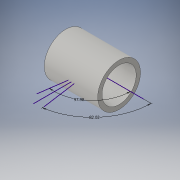
# Autodesk Inventor part: upper_arm_004
Saved by Autodesk Inventor 2016 SP1 (Build 200210100, 210)
## iProperties
Created: 2016-06-15
Part Number: upper_arm_004
Material: Generic
Document SubType Name: Modeling
Designer: asvsf
Density: 1 g/cm^3
Appearance: Default
Author: asvsf
Autodesk Inventor part; units mm, degrees
ref_plane "YZ Plane" through (0, 0, 0) normal (1, 0, 0) x (0, 1, 0)
ref_plane "XZ Plane" through (0, 0, 0) normal (0, 1, 0) x (-1, 0, 0)
ref_plane "XY Plane" through (0, 0, 0) normal (0, 0, 1) x (1, 0, 0)
sketch "Sketch1" plane through (0, 0, 0) normal (1, 0, 0) x (0, 1, 0)
  circle A0 centre (0, 0) radius 20
  circle A1 centre (0, 0) radius 16
  dimension "d0" = 40
  dimension "d1" = 32
  constraints: 2 centre point, 2 coincident
  measures "d0" diameter of A0
  measures "d1" diameter of A1
extrude "Extrusion1" add sketch "Sketch1" along normal mid plane 50
sketch "Sketch2" plane through (0, 0, 0) normal (0, 1, 0) x (-1, 0, 0)
  line L0 (0, 0) -> (6.4421, 45.9543)
  line L1 (0, 0) -> (-47.755, 0)
  line L2 (0, 0) -> (-7.3958, 52.7576)
  line L3 (0, 0) -> (0, 55.256)
  dimension "d4" = 97.98
  dimension "d5" = 82.02
  constraints: 8 end point, 1 horizontal, 1 vertical
  measures "d4" angle of L0 L1
  measures "d5" angle of L1 L2
body "Solid1"
